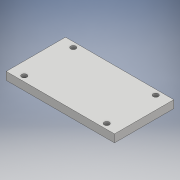
# Autodesk Inventor part: Деталь1
Saved by Autodesk Inventor 2018 (Build 220112000, 112)
## iProperties
Created: 2019-11-28
Part Number: Деталь1
Material: Типовые
Document SubType Name: Modeling
Designer: cosko
Density: 1 g/cm^3
Appearance: По умолчанию
Author: cosko
Autodesk Inventor part; units mm, degrees
ref_plane "YZ Plane" through (0, 0, 0) normal (1, 0, 0) x (0, 1, 0)
ref_plane "XZ Plane" through (0, 0, 0) normal (0, 1, 0) x (-1, 0, 0)
ref_plane "XY Plane" through (0, 0, 0) normal (0, 0, 1) x (1, 0, 0)
sketch "Эскиз1" plane through (0, 0, 0) normal (0, 0, 1) x (1, 0, 0)
  line L0 (-21, -11.5) -> (21, -11.5)
  line L1 (21, -11.5) -> (21, 11.5)
  line L2 (21, 11.5) -> (-21, 11.5)
  line L3 (-21, 11.5) -> (-21, -11.5)
  line L4 (-21, -11.5) -> (21, 11.5) construction
  line L5 (21, -11.5) -> (-21, 11.5) construction
  line L6 (21, -11.5) -> (16, -11.5) construction
  line L7 (16, -11.5) -> (16, -9.5) construction
  line L8 (-21, 11.5) -> (-16, 11.5) construction
  line L9 (-16, 11.5) -> (-16, 9.5) construction
  circle A0 centre (-16, 9.5) radius 1
  circle A1 centre (16, -9.5) radius 1
  line L10 (0, 11.5) -> (0, -11.5) construction
  circle A2 centre (16, 9.5) radius 1
  circle A3 centre (-16, -9.5) radius 1
  point P0 (0, 0)
  dimension "d0" = 42
  dimension "d1" = 23
  dimension "d2" = 5
  dimension "d3" = 2
  dimension "d4" = 5
  dimension "d5" = 2
  dimension "d6" = 2
  dimension "d7" = 2
  constraints: 22 end point, 4 centre point, 4 coincident, 4 midpoint, 4 symmetric about line, 3 perpendicular, 2 parallel, 2 point on line, 1 horizontal, 2 other
  measures "d0" distance of L2.end L1.end
  measures "d1" distance of L1.end L0.end
  measures "d2" distance of L0.end L6.end
  measures "d3" distance of L6.end L7.end
  measures "d4" distance of L2.end L8.end
  measures "d5" distance of L8.end L9.end
  measures "d6" diameter of A0
  measures "d7" diameter of A1
extrude "Выдавливание1" add sketch "Эскиз1" along normal blind 3
